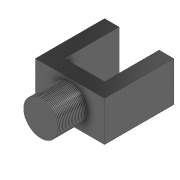
# Autodesk Inventor part: 09_Gripper
Saved by Autodesk Inventor 2022 (Build 260153000, 153)
## iProperties
Created: 2022-06-07
Part Number: 09_Gripper
Material: Generic
Document SubType Name: Modeling
Designer: pzach
Density: 1 g/cm^3
Appearance: Engine Turned
Author: pzach
Autodesk Inventor part; units mm, degrees
ref_plane "YZ Plane" through (0, 0, 0) normal (1, 0, 0) x (0, 1, 0)
ref_plane "XZ Plane" through (0, 0, 0) normal (0, 1, 0) x (-1, 0, 0)
ref_plane "XY Plane" through (0, 0, 0) normal (0, 0, 1) x (1, 0, 0)
sketch "Sketch2" plane through (0, 0, 0) normal (0, 0, 1) x (1, 0, 0)
  line L0 (-190, 110) -> (-110, 110)
  line L1 (-110, 110) -> (-110, -110)
  line L2 (-110, -110) -> (-190, -110)
  line L3 (-190, -110) -> (-190, 110)
  line L4 (-190, 110) -> (-110, -110) construction
  line L5 (-110, 110) -> (-190, -110) construction
  line L6 (0, 0) -> (0, 15) construction
  line L7 (190, 110) -> (110, 110)
  line L8 (110, 110) -> (110, -110)
  line L9 (110, -110) -> (190, -110)
  line L10 (190, -110) -> (190, 110)
  line L11 (190, 110) -> (110, -110) construction
  line L12 (110, 110) -> (190, -110) construction
  point P0 (-150, 0)
  point P1 (-150, 0)
  point P2 (150, 0)
  point P3 (150, 0)
  dimension "d0" = 80
  dimension "d1" = 220
  dimension "d2" = 150
  dimension "d3" = 15
  constraints: 26 end point, 6 symmetric about line, 5 midpoint, 2 parallel, 1 horizontal, 1 horizontal alignment, 1 perpendicular, 1 vertical
  measures "d0" distance of L0.start L0.end
  measures "d1" distance of L2.end L0.start
  measures "d2" distance of L6.start point (-150, 0)
  measures "d3" distance of L6.start L6.end
extrude "Extrusion1" add sketch "Sketch2" against normal blind 300
sketch "Sketch3" plane through (0, 0, 0) normal (0, 0, 1) x (1, 0, 0)
  line L0 (-190, 110) -> (-110, 110) projected
  line L1 (190, -110) -> (190, 110) projected
  line L2 (-190, 110) -> (190, 110)
  line L3 (190, 110) -> (190, -110)
  line L4 (190, -110) -> (-190, -110)
  line L5 (-190, -110) -> (-190, 110)
  point P0 (0, 0)
  constraints: 8 end point, 2 parallel, 1 horizontal, 1 perpendicular
extrude "Extrusion2" add sketch "Sketch3" along normal blind 80
sketch "Sketch4" plane through (0, 0, 80) normal (0, 0, 1) x (1, 0, 0)
  circle A0 centre (0, 0) radius 95
  dimension "d8" = 190
  constraints: 1 centre point, 1 coincident
  measures "d8" diameter of A0
extrude "Extrusion3" add sketch "Sketch4" along normal blind 160
thread "Thread1" size "M190x8" class "6g" standard "ANSI Metric M Profile" full length
body "Solid1"
